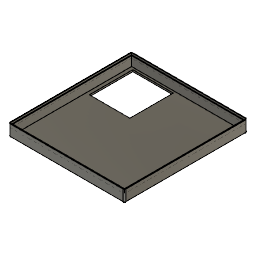
Casing Bottom (Autodesk Fusion 360 design; units mm, degrees)
part number: 2026-02-02-14-58-55-543
Autodesk Fusion 360 part; units mm, degrees
sketch "Sketch1" plane through (0, 0, 0) normal (0, 0, 1) x (1, 0, 0)
  line L0 (2, 0) -> (162, 0)
  line L1 (164, 2) -> (164, 172)
  line L2 (162, 174) -> (2, 174)
  line L3 (0, 172) -> (0, 2)
  arc A0 (2, 174) -> (0, 172) centre (2, 172) ccw
  arc A1 (164, 172) -> (162, 174) centre (162, 172) ccw
  arc A2 (0, 2) -> (2, 0) centre (2, 2) ccw
  arc A3 (162, 0) -> (164, 2) centre (162, 2) ccw
  point P0 (164, 0)
  point P1 (0, 174)
  dimension "d1" = 164
  dimension "d2" = 174
  dimension "d3" = 2
  dimension "d4" = 2
  dimension "d5" = 2
  dimension "d6" = 2
  constraint horizontal L0
  constraint vertical L1
  constraint horizontal L2
  constraint vertical L3
  constraint coincident P1 L2
  constraint coincident P1 L3
  constraint tangent L2 A0
  constraint tangent L3 A0
  constraint tangent L2 A1
  constraint tangent L1 A1
  constraint coincident origin L3
  constraint coincident origin L0
  constraint tangent L3 A2
  constraint tangent L0 A2
  constraint coincident P0 L1
  constraint coincident P0 L0
  constraint tangent L1 A3
  constraint tangent L0 A3
  measures "d1" distance of origin P0
  measures "d2" distance of origin P1
  measures "d3" radius of A0
  measures "d4" radius of A1
  measures "d5" radius of A2
  measures "d6" radius of A3
extrude "Extrude1" add sketch "Sketch1" along normal blind 17.5
sketch "Sketch2" plane through (0, 0, 17.5) normal (0, 0, 1) x (-1, 0, 0)
  arc A0 (-162, 0) -> (-164, -2) centre (-162, -2) ccw
  line L0 (-164, -2) -> (-164, -172)
  arc A1 (-164, -172) -> (-162, -174) centre (-162, -172) ccw
  line L1 (-162, -174) -> (-2, -174)
  arc A2 (-2, -174) -> (0, -172) centre (-2, -172) ccw
  line L2 (0, -172) -> (0, -2)
  arc A3 (0, -2) -> (-2, 0) centre (-2, -2) ccw
  line L3 (-2, 0) -> (-162, 0)
  line L4 (-1, -1) -> (-163, -1)
  line L5 (-163, -1) -> (-163, -173)
  line L6 (-163, -173) -> (-1, -173)
  line L7 (-1, -173) -> (-1, -1)
  dimension "d9" = 162
  dimension "d10" = 172
  dimension "d11" = 1
  dimension "d12" = 1
  constraint horizontal L4
  constraint vertical L5
  constraint horizontal L6
  constraint vertical L7
  measures "d9" distance of L4.start L4.end
  measures "d10" distance of L4.start L6.end
  measures "d11" distance of L2 L7
  measures "d12" distance of L3 L4
extrude "Extrude2" cut sketch "Sketch2" against normal blind 5 contours L4 L5 L6 L7
sketch "Sketch3" plane through (0, 0, 12.5) normal (0, 0, 1) x (-1, 0, 0)
  line L0 (-1, -173) -> (-1, -1)
  line L1 (-1, -1) -> (-163, -1)
  line L2 (-163, -1) -> (-163, -173)
  line L3 (-163, -173) -> (-1, -173)
  line L4 (-2, -172) -> (-162, -172)
  line L5 (-162, -172) -> (-162, -2)
  line L6 (-162, -2) -> (-2, -2)
  line L7 (-2, -2) -> (-2, -172)
  dimension "d15" = 160
  dimension "d16" = 170
  dimension "d17" = 1
  dimension "d18" = 1
  constraint horizontal L4
  constraint vertical L5
  constraint horizontal L6
  constraint vertical L7
  measures "d15" distance of L4.start L4.end
  measures "d16" distance of L4.start L6.end
  measures "d17" distance of L0 L7
  measures "d18" distance of L3 L4
extrude "Extrude3" add sketch "Sketch3" along normal blind 3.4 contours L4 L5 L6 L7
sketch "Sketch5" plane through (0, 0, 15.9) normal (0, 0, 1) x (-1, 0, 0)
  line L0 (-2, -2) -> (-162, -2)
  line L1 (-162, -2) -> (-162, -172)
  line L2 (-162, -172) -> (-2, -172)
  line L3 (-2, -172) -> (-2, -2)
  line L4 (-3, -171) -> (-161, -171)
  line L5 (-161, -171) -> (-161, -3)
  line L6 (-161, -3) -> (-3, -3)
  line L7 (-3, -3) -> (-3, -171)
  dimension "d27" = 158
  dimension "d28" = 168
  dimension "d29" = 1
  dimension "d30" = 1
  constraint horizontal L4
  constraint vertical L5
  constraint horizontal L6
  constraint vertical L7
  measures "d27" distance of L4.start L4.end
  measures "d28" distance of L4.start L6.end
  measures "d29" distance of L2 L4
  measures "d30" distance of L3 L7
extrude "Extrude5" cut sketch "Sketch5" against normal blind 13.4 contours L4 L5 L6 L7
sketch "Sketch6" plane through (0, 0, 2.5) normal (0, 0, 1) x (-1, 0, 0)
  line L0 (-3, -3) -> (-161, -3)
  line L1 (-161, -3) -> (-161, -171)
  line L2 (-161, -171) -> (-3, -171)
  line L3 (-3, -171) -> (-3, -3)
  line L4 (-7.765, -168.031) -> (-64.965, -168.031)
  line L5 (-64.965, -168.031) -> (-64.965, -106.731)
  line L6 (-64.965, -106.731) -> (-7.765, -106.731)
  line L7 (-7.765, -106.731) -> (-7.765, -168.031)
  line L8 (0, -172) -> (0, -2)
  line L9 (-162, -174) -> (-2, -174)
  dimension "d33" = 57.2
  dimension "d34" = 61.3
  dimension "d35" = 7.765
  dimension "d36" = 5.969
  constraint horizontal L4
  constraint vertical L5
  constraint horizontal L6
  constraint vertical L7
  measures "d33" distance of L4.start L4.end
  measures "d34" distance of L4.start L6.end
  measures "d35" distance of L7 L8
  measures "d36" distance of L4 L9
extrude "Extrude6" cut sketch "Sketch6" against normal blind 2.5 contours L4 L5 L6 L7
fillet "Fillet1" radius 2 8 edges at (163.4142, 173.4142, 0) (82, 174, 0) (0.5858, 173.4142, 0) (0, 87, 0) (0.5858, 0.5858, 0) (82, 0, 0) (163.4142, 0.5858, 0) (164, 87, 0)
